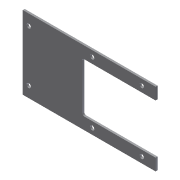
# Autodesk Inventor part: top support extension
Saved by Autodesk Inventor 2011 (Build 150239000, 239)
## iProperties
Created: 2011-06-09
Part Number: top support extension
Document SubType Name: Modeling
Designer: ijs09
Density: 1 g/cm^3
Author: ijs09
Autodesk Inventor part; units mm, degrees
ref_plane "YZ Plane" through (0, 0, 0) normal (1, 0, 0) x (0, 1, 0)
ref_plane "XZ Plane" through (0, 0, 0) normal (0, 1, 0) x (-1, 0, 0)
ref_plane "XY Plane" through (0, 0, 0) normal (0, 0, 1) x (1, 0, 0)
sketch "Sketch2" plane through (0, 0, 0) normal (0, 0, 1) x (1, 0, 0)
  line L0 (-40.3214, -37) -> (93.6786, -37)
  line L1 (93.6786, -37) -> (93.6786, -25)
  line L2 (93.6786, -25) -> (21.6786, -25)
  line L3 (19.6786, -23) -> (19.6786, 23)
  line L4 (21.6786, 25) -> (93.6786, 25)
  line L5 (93.6786, 25) -> (93.6786, 37)
  line L6 (93.6786, 37) -> (-40.3214, 37)
  line L7 (-40.3214, 37) -> (-40.3214, -37)
  arc A0 (21.6786, 25) -> (19.6786, 23) centre (21.6786, 23) ccw
  arc A1 (19.6786, -23) -> (21.6786, -25) centre (21.6786, -23) ccw
  circle A2 centre (-34.3214, 26) radius 2.15
  circle A3 centre (-34.3214, -26) radius 2.15
  circle A4 centre (29.6786, 31) radius 2.15
  circle A5 centre (79.6786, 31) radius 2.15
  circle A6 centre (79.6786, -31) radius 2.15
  circle A7 centre (29.6786, -31) radius 2.15
  point P0 (0, 0)
  dimension "d39" = 74
  dimension "d42" = 37
  dimension "d43" = 50
  dimension "d44" = 25
  dimension "d45" = 60
  dimension "d46" = 74
  dimension "d47" = 74
  dimension "d48" = 11
  dimension "d49" = 11
  dimension "d50" = 6
  dimension "d51" = 6
  dimension "d52" = 6
  dimension "d53" = 6
  dimension "d54" = 6
  dimension "d55" = 6
  dimension "d56" = 14
  dimension "d57" = 64
  dimension "d58" = 64
  dimension "d59" = 14
  dimension "d60" = 2
  dimension "d61" = 4.3
  dimension "d62" = 4.3
  dimension "d63" = 4.3
  dimension "d64" = 4.3
  dimension "d65" = 4.3
  dimension "d66" = 4.3
  dimension "d69" = 52
  constraints: 16 end point, 8 centre point, 6 coincident, 4 point on circle, 4 tangent, 3 parallel, 1 equal radius, 1 perpendicular
  measures "d39" distance between parallel lines of L0 L6
  measures "d42" distance from line of point (0, 0) L0
  measures "d43" distance between parallel lines of L2 L4
  measures "d44" distance from line of L2 point (0, 0)
  measures "d45" distance between parallel lines of L7 L3
  measures "d46" distance between parallel lines of L3 L5
  measures "d47" distance between parallel lines of L3 L1
  measures "d48" distance from line of L6 point (-34.321, 26)
  measures "d49" distance from line of L0 point (-34.321, -26)
  measures "d50" distance from line of L7 point (-34.321, -26)
  measures "d51" distance from line of L7 point (-34.321, 26)
  measures "d52" distance from line of L6 point (79.679, 31)
  measures "d53" distance from line of L6 point (29.679, 31)
  measures "d54" distance from line of L0 point (29.679, -31)
  measures "d55" distance from line of L0 point (79.679, -31)
  measures "d56" distance from line of point (79.679, 31) L5
  measures "d57" distance from line of point (29.679, 31) L5
  measures "d58" distance from line of point (29.679, -31) L1
  measures "d59" distance from line of point (79.679, -31) L1
  measures "d60" radius of A0
  measures "d61" diameter of A2
  measures "d62" diameter of A3
  measures "d63" diameter of A4
  measures "d64" diameter of A5
  measures "d65" diameter of A6
  measures "d66" diameter of A7
  measures "d69" distance of A3.centre A2.centre
extrude "Extrusion4" add sketch "Sketch2" along normal blind 2
equation "\"d42\" = 0.5 * d39"
equation "\"d44\" = 0.5 * d43"
equation "\"d62\" = d61"
equation "\"d63\" = d61"
equation "\"d64\" = d61"
equation "\"d65\" = d61"
equation "\"d66\" = d61"
body "Solid4"
